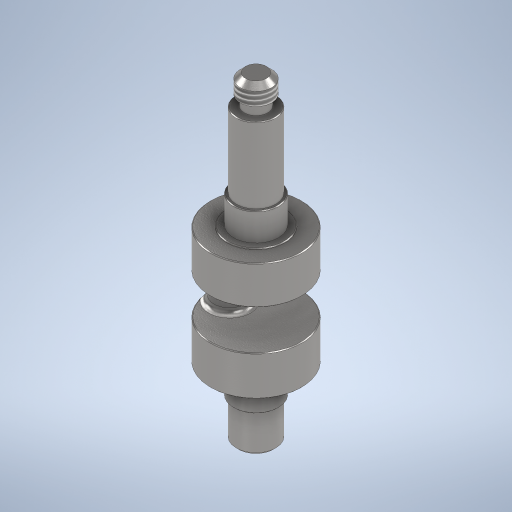
# Autodesk Inventor part: Exzenterwlle
Saved by Autodesk Inventor 2024 (Build 280153000, 153)
## iProperties
Created: 2024-03-01
Part Number: Exzenterwlle
Material: Stahl, galvanisiert
Document SubType Name: Modeling
Designer: ffogue
Density: 7.85 g/cm^3
Appearance: Galvanisiert
Author: ffogue
Autodesk Inventor part; units mm, degrees
ref_plane "YZ Plane" through (0, 0, 0) normal (1, 0, 0) x (0, 1, 0)
ref_plane "XZ Plane" through (0, 0, 0) normal (0, 1, 0) x (-1, 0, 0)
ref_plane "XY Plane" through (0, 0, 0) normal (0, 0, 1) x (1, 0, 0)
sketch "Skizze1" plane through (0, 0, 0) normal (0, 1, 0) x (-1, 0, 0)
  line L0 (10, -65) -> (10, -80)
  line L1 (10, -65) -> (16, -65)
  line L2 (16, -65) -> (16, -80)
  line L3 (16, -80) -> (10, -80)
  point P0 (0, 0)
  dimension "d52" = 65
  dimension "d53" = 15
  dimension "d54" = 12
  dimension "d81" = 10
  constraints: 8 end point, 2 perpendicular, 1 horizontal, 1 vertical
  measures "d52" vertical distance of point (0, 0) L0.start
  measures "d53" distance of L0.start L0.end
  measures "d54" diameter of L2 L0
  measures "d81" distance from line of point (0, 0) L0
sketch "Skizze5" plane through (0, 0, 0) normal (0, 1, 0) x (-1, 0, 0)
  line L0 (0, 0) -> (0, -65)
  line L1 (0, 0) -> (6, 0)
  line L2 (6, 0) -> (6, -7)
  line L3 (6, -7) -> (4.5, -7)
  line L4 (4.5, -7) -> (4.5, -11)
  line L5 (4.5, -11) -> (7.5, -11)
  line L6 (7.5, -11) -> (7.5, -39.5)
  line L7 (7.5, -39.5) -> (8.5, -39.5)
  line L8 (8.5, -39.5) -> (8.5, -50)
  line L9 (17.25, -50.5) -> (17.25, -65)
  line L10 (8.5, -50) -> (11, -50)
  line L11 (11, -50) -> (11, -50.5)
  line L12 (11, -50.5) -> (17.25, -50.5)
  line L13 (17.25, -65) -> (0, -65)
  point P0 (6, -11)
  dimension "d39" = 11
  dimension "d40" = 39.5
  dimension "d41" = 0.5
  dimension "d42" = 50
  dimension "d43" = 22
  dimension "d44" = 34.5
  dimension "d45" = 15
  dimension "d46" = 12
  dimension "d48" = 17
  dimension "d49" = 9
  dimension "d50" = 7
  dimension "d58" = 65
  constraints: 28 end point, 9 perpendicular, 3 horizontal, 1 midpoint
  measures "d39" distance from line of point (6, -11) L1
  measures "d40" distance between parallel lines of L1 L7
  measures "d41" distance between parallel lines of L12 L10
  measures "d42" distance between parallel lines of L1 L10
  measures "d43" diameter of L11 L0
  measures "d44" diameter of L9 L0
  measures "d45" diameter of L6 L0
  measures "d46" diameter of L2 L0
  measures "d48" diameter of L8 L0
  measures "d49" diameter of L4 L0
  measures "d50" distance between parallel lines of L3 L1
  measures "d58" distance between parallel lines of L1 L13
revolve "Umdrehung4" add sketch "Skizze1" angle 360 about axis through (-10, 0, -65) along (0, 0, -1)
revolve "Umdrehung5" add sketch "Skizze5" angle 360 about axis through (0, 0, 0) along (0, 0, -1)
sketch "Skizze6" plane through (0, 0, 0) normal (0, 1, 0) x (-1, 0, 0)
  line L0 (4, -80) -> (16, -80) projected
  line L1 (16.6064, -95) -> (11, -95)
  line L2 (11, -95) -> (11, -95.5)
  line L3 (11, -95.5) -> (8.5, -95.5)
  line L4 (8.5, -95.5) -> (8.5, -106)
  line L5 (8.5, -106) -> (7.5, -106)
  line L6 (7.5, -106) -> (7.5, -120.5)
  line L7 (7.5, -120.5) -> (0, -120.5)
  line L8 (0, -80) -> (0, -120.5)
  line L9 (0, -80) -> (17.25, -80)
  line L10 (17.25, -80) -> (17.25, -95)
  line L11 (17.25, -95) -> (16.6064, -95)
  point P0 (0, 0)
  point P1 (3.75, -120.5)
  dimension "d64" = 0.5
  dimension "d65" = 22
  dimension "d66" = 17
  dimension "d67" = 15
  dimension "d68" = 25
  dimension "d69" = 14.5
  dimension "d70" = 40.5
  dimension "d82" = 15
  dimension "d83" = 34.5
  constraints: 22 end point, 7 perpendicular, 1 collinear, 1 midpoint, 1 point on line, 1 vertical, 1 vertical alignment
  measures "d64" distance between parallel lines of L1 L3
  measures "d65" diameter of L2 L8
  measures "d66" diameter of L4 L8
  measures "d67" diameter of L6 L8
  measures "d68" vertical distance of L2.end point (3.75, -120.5)
  measures "d69" distance between parallel lines of L5 L7
  measures "d70" distance of L8.start L7.end
  measures "d82" distance of L9.end L10.end
  measures "d83" diameter of L10 L8
revolve "Umdrehung6" add sketch "Skizze6" angle 360 about axis through (0, 0, -80) along (0, 0, -1)
fillet "Rundung1" radius 2 1 edges at (-4, 0, -80)
chamfer "Fasen2" distance 1 angle 45 1 edges at (7.5, 0, -120.5)
chamfer "Fasen3" distance 2 angle 45 1 edges at (6, 0, 0)
thread "Gewinde1" size "M12x1.75" class "6g" standard "ISO Metric profile" full length
fillet "Rundung2" radius 2 1 edges at (-4, 0, -65)
chamfer "Fasen4" distance 0.3 angle 45 13 edges at (7.5, 0, -11) (8.5, 0, -39.5) (11, 0, -50) (17.25, 0, -50.5) (17.25, 0, -65) (-17.1056, 2.2271, -65.0781) (-17.1056, -2.2271, -65.0781) (17.25, 0, -80) (-17.1056, 2.2271, -79.9219) (-17.1056, -2.2271, -79.9219) (17.25, 0, -95) (11, 0, -95.5) (8.5, 0, -106)
